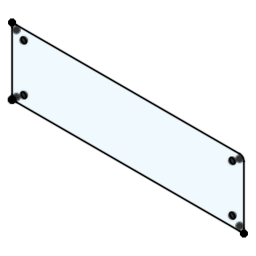
BeoMasterBlende (Autodesk Fusion 360 design; units mm, degrees)
Autodesk Fusion 360 part; units mm, degrees
sketch "Skizze1" plane through (0, 0, 0) normal (0, 1, 0) x (1, 0, 0)
  line L0 (0, 0) -> (140, 0)
  line L1 (140, 0) -> (140, -46)
  line L2 (140, -46) -> (0, -46)
  line L3 (0, -46) -> (0, 0)
  circle A0 centre (4, -42) radius 1.6
  circle A1 centre (4, -4) radius 1.6
  circle A2 centre (136, -42) radius 1.6
  circle A3 centre (136, -4) radius 1.6
  line L4 (10, -36.5) -> (130, -36.5)
  line L5 (130, -36.5) -> (130, -9.5)
  line L6 (130, -9.5) -> (10, -9.5)
  line L7 (10, -9.5) -> (10, -36.5)
  line L8 (11, -36.65) -> (62.2, -36.65)
  line L9 (62.2, -36.65) -> (62.2, -9.35)
  line L10 (62.2, -9.35) -> (11, -9.35)
  line L11 (11, -9.35) -> (11, -36.65)
  line L12 (77.8, -36.65) -> (129, -36.65)
  line L13 (129, -36.65) -> (129, -9.35)
  line L14 (129, -9.35) -> (77.8, -9.35)
  line L15 (77.8, -9.35) -> (77.8, -36.65)
  circle A4 centre (13.8, -33.85) radius 1.05
  circle A5 centre (59.4, -33.85) radius 1.05
  circle A6 centre (13.8, -12.15) radius 1.05
  circle A7 centre (59.4, -12.15) radius 1.05
  circle A8 centre (80.6, -33.85) radius 1.05
  circle A9 centre (80.6, -12.15) radius 1.05
  circle A10 centre (126.2, -33.85) radius 1.05
  circle A11 centre (126.2, -12.15) radius 1.05
  line L16 (8, -31.1) -> (132, -31.1)
  line L17 (132, -31.1) -> (132, -15.1)
  line L18 (132, -15.1) -> (8, -15.1)
  line L19 (8, -15.1) -> (8, -31.1)
  circle A12 centre (7, -36) radius 1.6
  circle A13 centre (133, -10) radius 1.6
  circle A14 centre (133, -36) radius 1.6
  circle A15 centre (7, -10) radius 1.6
  dimension "d1" = 140
  dimension "d2" = 46
  dimension "d3" = 3.2
  dimension "d4" = 3.2
  dimension "d5" = 3.2
  dimension "d6" = 3.2
  dimension "d7" = 132
  dimension "d8" = 38
  dimension "d9" = 38
  dimension "d10" = 132
  dimension "d11" = 4
  dimension "d12" = 4
  dimension "d60" = 120
  dimension "d61" = 27
  dimension "d62" = 9.5
  dimension "d63" = 10
  dimension "d64" = 1
  dimension "d65" = 1
  dimension "d66" = 51.2
  dimension "d67" = 51.2
  dimension "d68" = 27.3
  dimension "d69" = 27.3
  dimension "d70" = 0.15
  dimension "d71" = 0.15
  dimension "d72" = 2.1
  dimension "d73" = 2.1
  dimension "d74" = 2.1
  dimension "d75" = 2.1
  dimension "d76" = 2.1
  dimension "d77" = 2.1
  dimension "d78" = 2.1
  dimension "d79" = 2.1
  dimension "d80" = 2.8
  dimension "d81" = 2.8
  dimension "d82" = 2.8
  dimension "d83" = 2.8
  dimension "d84" = 45.6
  dimension "d85" = 45.6
  dimension "d86" = 21.7
  dimension "d87" = 21.7
  dimension "d88" = 45.6
  dimension "d89" = 21.7
  dimension "d90" = 21.7
  dimension "d91" = 16
  dimension "d92" = 124
  dimension "d95" = 5.55
  dimension "d115" = 3.2
  dimension "d116" = 3.2
  dimension "d117" = 3.2
  dimension "d118" = 3.2
  dimension "d121" = 126
  dimension "d123" = 10
  dimension "d124" = 7
  dimension "d125" = 26
  dimension "d126" = 126
  dimension "d127" = 26
  dimension "d128" = 36
  dimension "d129" = 133
  dimension "d130" = 133
  dimension "d131" = 8
  constraint horizontal L0
  constraint vertical L1
  constraint horizontal L2
  constraint vertical L3
  constraint coincident L0.start L3.end
  constraint horizontal L4
  constraint vertical L5
  constraint horizontal L6
  constraint vertical L7
  constraint horizontal L8
  constraint vertical L9
  constraint horizontal L10
  constraint vertical L11
  constraint horizontal L12
  constraint vertical L13
  constraint horizontal L14
  constraint vertical L15
  constraint vertical A4.centre A6.centre
  constraint horizontal A4.centre A5.centre
  constraint horizontal A8.centre A10.centre
  constraint vertical A8.centre A9.centre
  constraint vertical A10.centre A11.centre
  constraint vertical A0.centre A1.centre
  constraint horizontal A0.centre A2.centre
  constraint horizontal L16
  constraint vertical L17
  constraint horizontal L18
  constraint vertical L19
  measures "d1" distance of L0.start L0.end
  measures "d2" distance of L0.start L2.end
  measures "d3" diameter of A0
  measures "d4" diameter of A1
  measures "d5" diameter of A2
  measures "d6" diameter of A3
  measures "d7" distance of A0.centre A2.centre
  measures "d8" distance of A0.centre A1.centre
  measures "d9" vertical distance of A2.centre A3.centre
  measures "d10" distance of A1.centre A3.centre
  measures "d11" distance of L2 A0.centre
  measures "d12" distance of L3 A0.centre
  measures "d60" distance of L4.start L4.end
  measures "d61" distance of L4.start L6.end
  measures "d62" distance of L0 L6
  measures "d63" distance of L3 L7
  measures "d64" distance of L5 L13
  measures "d65" distance of L7 L11
  measures "d66" distance of L8.start L8.end
  measures "d67" distance of L12.start L12.end
  measures "d68" distance of L12.start L14.end
  measures "d69" distance of L8.end L9.end
  measures "d70" distance of L4 L8
  measures "d71" distance of L4 L12
  measures "d72" diameter of A4
  measures "d73" diameter of A5
  measures "d74" diameter of A6
  measures "d75" diameter of A7
  measures "d76" diameter of A8
  measures "d77" diameter of A9
  measures "d78" diameter of A10
  measures "d79" diameter of A11
  measures "d80" distance of L11 A4.centre
  measures "d81" distance of L8 A4.centre
  measures "d82" distance of L15 A8.centre
  measures "d83" distance of L12 A8.centre
  measures "d84" distance of A4.centre A5.centre
  measures "d85" horizontal distance of A6.centre A7.centre
  measures "d86" vertical distance of A4.centre A6.centre
  measures "d87" vertical distance of A5.centre A7.centre
  measures "d88" distance of A8.centre A10.centre
  measures "d89" distance of A8.centre A9.centre
  measures "d90" distance of A10.centre A11.centre
  measures "d91" distance of L16.end L17.end
  measures "d92" distance of L17 L19
  measures "d95" distance of L8 L16
  measures "d115" diameter of A12
  measures "d116" diameter of A15
  measures "d117" diameter of A14
  measures "d118" diameter of A13
  measures "d121" distance of A15.centre A13.centre
  measures "d123" distance of L0 A15.centre
  measures "d124" distance of L3 A15.centre
  measures "d125" distance of A15.centre A12.centre
  measures "d126" distance of A14.centre A12.centre
  measures "d127" distance of A14.centre A13.centre
  measures "d128" distance of L0 A12.centre
  measures "d129" distance of L3 A13.centre
  measures "d130" distance of L3 A14.centre
  measures "d131" distance of L3 L19
extrude "Extrusion1" add sketch "Skizze1" along normal blind 3 contours L0 L1 L2 L3 | L4 L7 L11 L16 | L4 L9 L11 L16 | L4 L8 L9 L11 | L7 L16 L18 L19 | L7 L11 L16 L18 | L4 L9 L15 L16 | L9 L11 L16 L18 | L6 L7 L11 L18 | L4 L13 L15 L16 | L4 L12 L13 L15 | L9 L15 L16 L18 | L6 L9 L11 L18 | L4 L5 L13 L16 | L13 L15 L16 L18 | L6 L9 L15 L18 | L6 L9 L10 L11 | L5 L13 L16 L18 | L6 L13 L15 L18 | L5 L16 L17 L18 | L5 L6 L13 L18 | L6 L13 L14 L15 | A4 | A5 | A6 | A7 | A8 | A9 | A10 | A11 | A12 | A13 | A14 | A15
sketch "Skizze4" plane through (0, 0, 0) normal (0, 1, 0) x (1, 0, 0)
  line L0 (7, -39) -> (133, -39)
  line L1 (133, -33) -> (133, -13)
  line L2 (133, -7) -> (7, -7)
  line L3 (7, -13) -> (7, -33)
  arc A0 (7, -33) -> (7, -39) centre (7, -36) ccw
  arc A1 (133, -13) -> (133, -7) centre (133, -10) ccw
  arc A2 (133, -39) -> (133, -33) centre (133, -36) ccw
  arc A3 (7, -7) -> (7, -13) centre (7, -10) ccw
  circle A4 centre (7, -36) radius 1.6
  circle A5 centre (7, -10) radius 1.6
  circle A6 centre (133, -36) radius 1.6
  circle A7 centre (133, -10) radius 1.6
  dimension "d99" = 126
  dimension "d100" = 32
  dimension "d101" = 6
  dimension "d102" = 3
  dimension "d103" = 6
  dimension "d104" = 6
  dimension "d105" = 6
  dimension "d106" = 3
  dimension "d107" = 3
  dimension "d108" = 3
  dimension "d109" = 7
  dimension "d110" = 7
  dimension "d111" = 3.2
  dimension "d112" = 3.2
  dimension "d113" = 3.2
  dimension "d114" = 3.2
  constraint horizontal L0
  constraint vertical L1
  constraint horizontal L2
  constraint vertical L3
  constraint coincident L3 A0.centre
  constraint coincident L3 A3.centre
  constraint coincident L1 A2.centre
  constraint coincident L1 A1.centre
  constraint concentric A0 A4
  constraint concentric A3 A5
  constraint concentric A2 A6
  constraint concentric A1 A7
  measures "d99" distance of L2.start L2.end
  measures "d100" distance of L0.end L2.start
  measures "d101" diameter of A0
  measures "d102" distance of L0 A0.centre
  measures "d103" diameter of A3
  measures "d104" diameter of A2
  measures "d105" diameter of A1
  measures "d106" distance of L2 A3.centre
  measures "d107" distance of L0 A2.centre
  measures "d108" distance of L2 A1.centre
  measures "d109" distance of origin L2
  measures "d110" distance of origin L3
  measures "d111" diameter of A4
  measures "d112" diameter of A5
  measures "d113" diameter of A6
  measures "d114" diameter of A7
sketch "Skizze5" plane through (0, 0, 0) normal (0, 1, 0) x (1, 0, 0)
  line L0 (7, -39) -> (133, -39)
  arc A0 (7, -33) -> (7, -39) centre (7, -36) ccw
  line L1 (7, -13) -> (7, -33)
  arc A1 (7, -7) -> (7, -13) centre (7, -10) ccw
  line L2 (133, -7) -> (7, -7)
  arc A2 (133, -13) -> (133, -7) centre (133, -10) ccw
  line L3 (133, -33) -> (133, -13)
  arc A3 (133, -39) -> (133, -33) centre (133, -36) ccw
  line L4 (77.8, -9.35) -> (77.8, -36.65)
  line L5 (77.8, -36.65) -> (129, -36.65)
  line L6 (129, -36.65) -> (129, -9.35)
  line L7 (129, -9.35) -> (77.8, -9.35)
  line L8 (62.2, -9.35) -> (11, -9.35)
  line L9 (62.2, -36.65) -> (62.2, -9.35)
  line L10 (11, -9.35) -> (11, -36.65)
  line L11 (11, -36.65) -> (62.2, -36.65)
  line L12 (17.25, -34.35) -> (59.97, -34.35)
  line L13 (59.97, -34.35) -> (59.97, -11.65)
  line L14 (59.97, -11.65) -> (17.25, -11.65)
  line L15 (17.25, -11.65) -> (17.25, -34.35)
  line L16 (122.75, -34.35) -> (80.03, -34.35)
  line L17 (80.03, -34.35) -> (80.03, -11.65)
  line L18 (80.03, -11.65) -> (122.75, -11.65)
  line L19 (122.75, -11.65) -> (122.75, -34.35)
  dimension "d132" = 126
  dimension "d133" = 32
  dimension "d134" = 6
  dimension "d135" = 3
  dimension "d136" = 6
  dimension "d137" = 6
  dimension "d138" = 6
  dimension "d139" = 3
  dimension "d140" = 3
  dimension "d141" = 3
  dimension "d142" = 51.2
  dimension "d143" = 51.2
  dimension "d144" = 27.3
  dimension "d145" = 27.3
  dimension "d146" = 7
  dimension "d147" = 7
  dimension "d148" = 9.35
  dimension "d149" = 9.35
  dimension "d150" = 11
  dimension "d151" = 77.8
  dimension "d152" = 6.25
  dimension "d153" = 6.25
  dimension "d154" = 2.23
  dimension "d155" = 2.23
  dimension "d156" = 2.3
  dimension "d157" = 2.3
  dimension "d158" = 2.3
  dimension "d159" = 2.3
  constraint horizontal L0
  constraint vertical L3
  constraint horizontal L2
  constraint vertical L1
  constraint coincident A0.centre L1
  constraint coincident A1.centre L1
  constraint coincident A3.centre L3
  constraint coincident A2.centre L3
  constraint horizontal L11
  constraint vertical L9
  constraint horizontal L8
  constraint vertical L10
  constraint horizontal L5
  constraint vertical L6
  constraint horizontal L7
  constraint vertical L4
  constraint horizontal L12
  constraint vertical L13
  constraint horizontal L14
  constraint vertical L15
  constraint horizontal L16
  constraint vertical L17
  constraint horizontal L18
  constraint vertical L19
  measures "d132" distance of L2.start A1.start
  measures "d133" distance of L2.start L0.end
  measures "d134" diameter of A0
  measures "d135" distance of A0.centre L0
  measures "d136" diameter of A1
  measures "d137" diameter of A3
  measures "d138" diameter of A2
  measures "d139" distance of A1.centre L2
  measures "d140" distance of A3.centre L0
  measures "d141" distance of A2.centre L2
  measures "d142" distance of L9.start L10.end
  measures "d143" distance of L5.end L4.end
  measures "d144" distance of L4.end L4.start
  measures "d145" distance of L9.start L8.start
  measures "d146" distance of origin L2
  measures "d147" distance of origin L1
  measures "d148" distance of origin L8
  measures "d149" distance of origin L7
  measures "d150" distance of origin L10
  measures "d151" distance of origin L4
  measures "d152" distance of L10 L15
  measures "d153" distance of L6 L19
  measures "d154" distance of L9 L13
  measures "d155" distance of L4 L17
  measures "d156" distance of L11 L12
  measures "d157" distance of L8 L14
  measures "d158" distance of L5 L16
  measures "d159" distance of L7 L18
sketch "Skizze6" plane through (0, 0, 0) normal (0, 1, 0) x (1, 0, 0)
  line L0 (4, 0) -> (211, 0)
  line L1 (215, -4) -> (215, -58)
  line L2 (211, -62) -> (4, -62)
  line L3 (0, -58) -> (0, -4)
  circle A0 centre (10.75, -53) radius 2.25
  circle A1 centre (10.75, -9) radius 2.25
  circle A2 centre (204.25, -53) radius 2.25
  circle A3 centre (204.25, -9) radius 2.25
  arc A4 (0, -58) -> (4, -62) centre (4, -58) ccw
  arc A5 (4, 0) -> (0, -4) centre (4, -4) ccw
  arc A6 (211, -62) -> (215, -58) centre (211, -58) ccw
  arc A7 (215, -4) -> (211, 0) centre (211, -4) ccw
  point P0 (215, 0)
  point P1 (0, -62)
  dimension "d160" = 62
  dimension "d161" = 215
  dimension "d162" = 4.5
  dimension "d163" = 4.5
  dimension "d164" = 4.5
  dimension "d165" = 4.5
  dimension "d167" = 193.5
  dimension "d168" = 44
  dimension "d170" = 9
  dimension "d171" = 10.75
  dimension "d172" = 4
  dimension "d173" = 4
  dimension "d174" = 4
  dimension "d175" = 4
  constraint horizontal L0
  constraint vertical L1
  constraint horizontal L2
  constraint vertical L3
  constraint vertical A0.centre A1.centre
  constraint horizontal A1.centre A3.centre
  constraint horizontal A0.centre A2.centre
  constraint vertical A2.centre A3.centre
  constraint coincident P1 L2
  constraint coincident P1 L3
  constraint tangent L2 A4
  constraint tangent L3 A4
  constraint coincident origin L0
  constraint coincident origin L3
  constraint tangent L0 A5
  constraint tangent L3 A5
  constraint tangent L1 A6
  constraint tangent L2 A6
  constraint coincident P0 L0
  constraint coincident P0 L1
  constraint tangent L0 A7
  constraint tangent L1 A7
  measures "d160" distance of origin P1
  measures "d161" distance of origin P0
  measures "d162" diameter of A0
  measures "d163" diameter of A1
  measures "d164" diameter of A2
  measures "d165" diameter of A3
  measures "d167" distance of A1.centre A3.centre
  measures "d168" distance of A0.centre A1.centre
  measures "d170" distance of L0 A1.centre
  measures "d171" distance of L3 A1.centre
  measures "d172" radius of A4
  measures "d173" radius of A5
  measures "d174" radius of A6
  measures "d175" radius of A7
